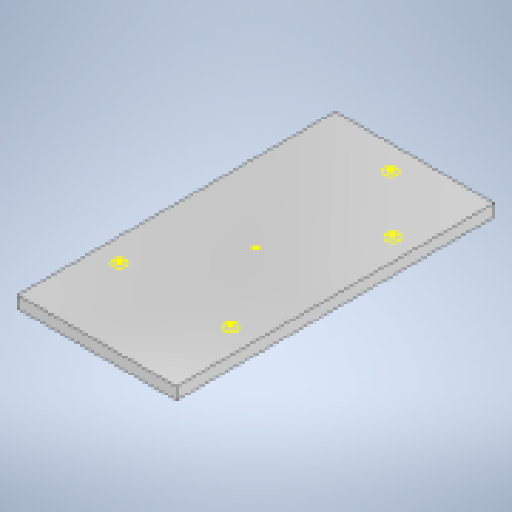
# Autodesk Inventor part: axis_22_top_frame(middle)
Saved by Autodesk Inventor 2025.2 (Build 292293000, 293)
## iProperties
Created: 2025-05-07
Part Number: axis_22_top_frame(middle)
Material: Aluminum 6061-AHC
Document SubType Name: Sheet Metal
Designer: LG
Density: 2.7 g/cm^3
Sheet Metal Rule: Default_mm
Appearance: Aluminum - Dark
Author: LG
Autodesk Inventor part; units mm, degrees
ref_plane "YZ Plane" through (0, 0, 0) normal (1, 0, 0) x (0, 1, 0)
ref_plane "XZ Plane" through (0, 0, 0) normal (0, 1, 0) x (-1, 0, 0)
ref_plane "XY Plane" through (0, 0, 0) normal (0, 0, 1) x (1, 0, 0)
sketch "Sketch1" plane through (0, 0, 0) normal (0, 1, 0) x (-1, 0, 0)
  line L0 (-10, 20) -> (10, 20)
  line L1 (10, 20) -> (10, -20)
  line L2 (10, -20) -> (-10, -20)
  line L3 (-10, -20) -> (-10, 20)
  line L4 (-10, 20) -> (10, -20) construction
  line L5 (10, 20) -> (-10, -20) construction
  point P0 (0, 0)
  dimension "d0" = 40
  dimension "d1" = 20
  measures "d0" distance of L0.end L1.end
  measures "d1" distance of L1.end L2.end
extrude "Plate1" add sketch "Sketch1" along normal blind 1.5
sketch "Sketch2" plane through (0, 1.5, 0) normal (0, 1, 0) x (1, 0, 0)
  circle A0 centre (7.32, 9.93) radius 0.7835 projected
  circle A1 centre (0.02, 16.93) radius 0.7835 projected
  circle A2 centre (6.93, -10.12) radius 0.7835 projected
  circle A3 centre (-7.07, -10.12) radius 0.7835 projected
  point P0 (0, 0)
sketch "Sketch3" plane through (0, 1.5, 0) normal (0, 1, 0) x (1, 0, 0)
  circle A0 centre (0.02, 2.93) radius 0.7835 projected
  line L0 (10, 20) -> (10, -20) projected
  line L1 (-10, 20) -> (10, 20) projected
  line L2 (-10, -20) -> (-10, 20) projected
  line L3 (10, -20) -> (-10, -20) projected
  circle A1 centre (-7.595, -17.74) radius 0.7835 projected
  circle A2 centre (7.455, -17.74) radius 0.7835 projected
  point P0 (0, 0)
hole "Hole1" at (0.02, 1.5, -16.93) at (7.32, 1.5, -9.93) at (6.93, 1.5, 10.12) at (-7.07, 1.5, 10.12) direction (0, -1, 0) diameter 2.1 depth 1.5
hole "Hole2" at (7.455, 1.5, 17.74) at (-7.595, 1.5, 17.74) at (0.02, 1.5, -2.93) direction (0, -1, 0) diameter 2.1 depth 1.5
equation "\"d8\" = Thickness"
equation "\"d15\" = Thickness"
equation "\"d2\" = Thickness"
equation "\"BendReliefWidth\" = Thickness"
equation "\"BendReliefDepth\" = 0.5 * Thickness"
equation "\"CornerReliefSize\" = 4 * Thickness"
equation "\"MinimumRemnant\" = 2 * Thickness"
equation "\"TransitionRadius\" = BendRadius"
equation "\"JacobiRadiusSize\" = BendRadius"
equation "\"GapSize\" = Thickness"
equation "\"Thickness\" = 1.5"
equation "\"BendRadius\" = 0.31"
body "Solid1"
